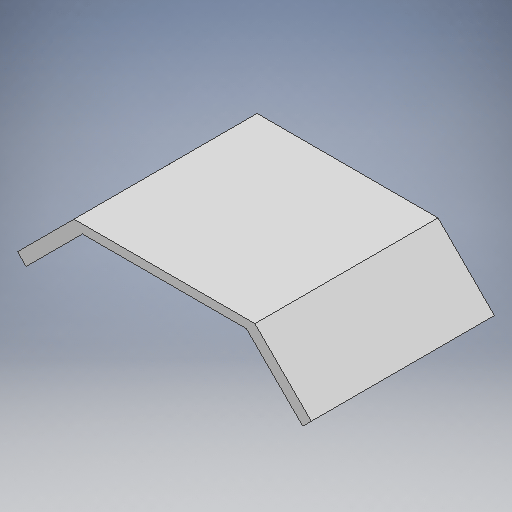
# Autodesk Inventor part: 1ipt
Saved by Autodesk Inventor 2025.2 (Build 292293000, 293)
## iProperties
Created: 2025-03-17
Part Number: 1ipt
Material: 일반
Document SubType Name: Modeling
Designer: jbhma
Density: 1 g/cm^3
Appearance: 기본값
Author: jbhma
Autodesk Inventor part; units mm, degrees
ref_plane "YZ Plane" through (0, 0, 0) normal (1, 0, 0) x (0, 1, 0)
ref_plane "XZ Plane" through (0, 0, 0) normal (0, 1, 0) x (-1, 0, 0)
ref_plane "XY Plane" through (0, 0, 0) normal (0, 0, 1) x (1, 0, 0)
sketch "스케치1" plane through (0, 0, 0) normal (0, 1, 0) x (-1, 0, 0)
  line L0 (0, 0) -> (-420, 0)
  line L1 (-420, 0) -> (-420, -425)
  line L2 (-420, -425) -> (0, -425)
  line L3 (0, -425) -> (0, 0)
  dimension "d0" = 420
  dimension "d1" = 425
  constraints: 8 end point, 2 parallel, 1 horizontal, 1 perpendicular
  measures "d0" distance of L2.end L1.end
  measures "d1" distance of L1.end L0.end
extrude "돌출1" add sketch "스케치1" along normal blind 20
chamfer "모따기1" distance 20 angle 45 1 edges at (420, 0, -212.5)
chamfer "모따기2" distance 20 angle 45 1 edges at (0, 0, -212.5)
sketch "스케치9" plane through (420, 20, 0) normal (0.7071068, -0.7071068, 0) x (-0.7071068, -0.7071068, 0)
  line L0 (0, 0) -> (28, 0)
  line L1 (28, 0) -> (28, 425)
  line L2 (28, 425) -> (0, 425)
  line L3 (0, 425) -> (0, 0)
  point P0 (311.127, 0)
  constraints: 8 end point, 2 parallel, 1 horizontal, 1 perpendicular
sketch "스케치10" plane through (0, 20, 0) normal (-0.7071068, -0.7071068, 0) x (-0.7071068, 0.7071068, 0)
  line L0 (0, 425) -> (-28, 425)
  line L1 (-28, 425) -> (-28, 0)
  line L2 (-28, 0) -> (0, 0)
  line L3 (0, 0) -> (0, 425)
  point P0 (-14.1421, 0)
  constraints: 8 end point, 2 parallel, 1 horizontal, 1 perpendicular
extrude "돌출2" add sketch "스케치10" along normal blind 185
extrude "돌출3" add sketch "스케치9" along normal blind 185
